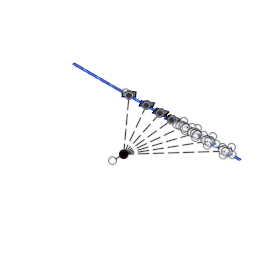
Sonar_bracket_alignment_thingy v7 (Autodesk Fusion 360 design; units mm, degrees)
Autodesk Fusion 360 part; units mm, degrees
note: some values were not read from the file. Set by a fixed rule: which sketch regions a step uses.
sketch "Sketch1" plane through (0, 0, 0) normal (0, 1, 0) x (1, 0, 0)
  line L0 (0, 0) -> (31.2124, 296.9662) construction
  line L1 (0, 0) -> (96.3772, 296.6185) construction
  line L2 (0, 0) -> (170.86, 295.9383) construction
  line L3 (0, 0) -> (265.5789, 294.9552) construction
  line L4 (0, 0) -> (0, -60) construction
  line L5 (0, 0) -> (-31.2124, 296.9662) construction
  line L6 (0, 0) -> (-170.86, 295.9383) construction
  line L7 (0, 0) -> (-265.5789, 294.9552) construction
  line L8 (0, 0) -> (-96.3772, 296.6185) construction
  line L9 (-257.5953, 325.6922) -> (-296.982, 290.2283)
  line L10 (-296.982, 290.2283) -> (-273.5624, 264.2182)
  line L11 (-273.5624, 264.2182) -> (-234.1758, 299.6822)
  line L12 (-234.1758, 299.6822) -> (-257.5953, 325.6922)
  line L13 (-257.5953, 325.6922) -> (-273.5624, 264.2182) construction
  line L14 (-296.982, 290.2283) -> (-234.1758, 299.6822) construction
  line L15 (-156.6604, 324.3437) -> (-202.5597, 297.8437)
  line L16 (-202.5597, 297.8437) -> (-185.0597, 267.5328)
  line L17 (-185.0597, 267.5328) -> (-139.1604, 294.0328)
  line L18 (-139.1604, 294.0328) -> (-156.6604, 324.3437)
  line L19 (-156.6604, 324.3437) -> (-185.0597, 267.5328) construction
  line L20 (-76.582, 321.451) -> (-126.988, 305.0731)
  line L21 (-126.988, 305.0731) -> (-116.1724, 271.7861)
  line L22 (-116.1724, 271.7861) -> (-65.7664, 288.164)
  line L23 (-65.7664, 288.164) -> (-76.582, 321.451)
  line L24 (-76.582, 321.451) -> (-116.1724, 271.7861) construction
  line L25 (-126.988, 305.0731) -> (-65.7664, 288.164) construction
  line L26 (-6.6868, 317.1404) -> (-59.3965, 311.6004)
  line L27 (-59.3965, 311.6004) -> (-55.738, 276.7921)
  line L28 (-55.738, 276.7921) -> (-3.0283, 282.3321)
  line L29 (-3.0283, 282.3321) -> (-6.6868, 317.1404)
  line L30 (-6.6868, 317.1404) -> (-55.738, 276.7921) construction
  line L31 (-59.3965, 311.6004) -> (-3.0283, 282.3321) construction
  line L32 (3.0283, 282.3321) -> (6.6868, 317.1404)
  line L33 (6.6868, 317.1404) -> (59.3965, 311.6004)
  line L34 (55.738, 276.7921) -> (3.0283, 282.3321)
  line L35 (59.3965, 311.6004) -> (55.738, 276.7921)
  line L36 (116.1724, 271.7861) -> (65.7664, 288.164)
  line L37 (65.7664, 288.164) -> (76.582, 321.451)
  line L38 (76.582, 321.451) -> (126.988, 305.0731)
  line L39 (126.988, 305.0731) -> (116.1724, 271.7861)
  line L40 (139.1604, 294.0328) -> (156.6604, 324.3437)
  line L41 (156.6604, 324.3437) -> (202.5597, 297.8437)
  line L42 (202.5597, 297.8437) -> (185.0597, 267.5328)
  line L43 (185.0597, 267.5328) -> (139.1604, 294.0328)
  line L44 (273.5624, 264.2182) -> (234.1758, 299.6822)
  line L45 (234.1758, 299.6822) -> (257.5953, 325.6922)
  line L46 (257.5953, 325.6922) -> (296.982, 290.2283)
  line L47 (296.982, 290.2283) -> (273.5624, 264.2182)
  line L48 (-258.5243, 324.8558) -> (-296.0531, 291.0647)
  line L49 (-296.0531, 291.0647) -> (-272.6335, 265.0547)
  line L50 (-272.6335, 265.0547) -> (-235.1047, 298.8457)
  line L51 (-235.1047, 298.8457) -> (-258.5243, 324.8558)
  line L52 (-258.5243, 324.8558) -> (-272.6335, 265.0547) construction
  line L53 (-296.0531, 291.0647) -> (-235.1047, 298.8457) construction
  line L54 (-157.7429, 323.7187) -> (-201.4772, 298.4687)
  line L55 (-201.4772, 298.4687) -> (-183.9772, 268.1578)
  line L56 (-183.9772, 268.1578) -> (-140.2429, 293.4078)
  line L57 (-140.2429, 293.4078) -> (-157.7429, 323.7187)
  line L58 (-157.7429, 323.7187) -> (-183.9772, 268.1578) construction
  line L59 (-201.4772, 298.4687) -> (-140.2429, 293.4078) construction
  line L60 (-77.7708, 321.0647) -> (-125.7992, 305.4593)
  line L61 (-125.7992, 305.4593) -> (-114.9836, 272.1724)
  line L62 (-114.9836, 272.1724) -> (-66.9552, 287.7777)
  line L63 (-66.9552, 287.7777) -> (-77.7708, 321.0647)
  line L64 (-77.7708, 321.0647) -> (-114.9836, 272.1724) construction
  line L65 (-125.7992, 305.4593) -> (-66.9552, 287.7777) construction
  line L66 (-7.93, 317.0097) -> (-58.1533, 311.731)
  line L67 (-58.1533, 311.731) -> (-54.4948, 276.9228)
  line L68 (-54.4948, 276.9228) -> (-4.2715, 282.2015)
  line L69 (-4.2715, 282.2015) -> (-7.93, 317.0097)
  line L70 (-7.93, 317.0097) -> (-54.4948, 276.9228) construction
  line L71 (-58.1533, 311.731) -> (-4.2715, 282.2015) construction
  line L72 (296.0531, 291.0647) -> (272.6335, 265.0547)
  line L73 (235.1047, 298.8457) -> (258.5243, 324.8558)
  line L74 (201.4772, 298.4687) -> (183.9772, 268.1578)
  line L75 (140.2429, 293.4078) -> (157.7429, 323.7187)
  line L76 (125.7992, 305.4593) -> (114.9836, 272.1724)
  line L77 (66.9552, 287.7777) -> (77.7708, 321.0647)
  line L78 (58.1533, 311.731) -> (54.4948, 276.9228)
  line L79 (4.2715, 282.2015) -> (7.93, 317.0097)
  line L80 (340.5789, 293.5101) -> (-559.4211, 293.5101)
  line L81 (-559.4211, 293.5101) -> (-559.4211, 284.5101)
  line L82 (-559.4211, 284.5101) -> (340.5789, 284.5101)
  line L83 (340.5789, 284.5101) -> (340.5789, 293.5101)
  line L84 (340.5789, 293.5101) -> (-559.4211, 284.5101) construction
  line L85 (-559.4211, 293.5101) -> (340.5789, 284.5101) construction
  line L86 (-257.6212, 293.5101) -> (-282.6212, 293.5101)
  line L87 (-559.4211, 289.0101) -> (340.5789, 289.0101) construction
  circle A0 centre (-260.2258, 289.0101) radius 3.5
  line L88 (-272.7258, 293.5101) -> (-247.7258, 293.5101)
  line L89 (-247.7258, 293.5101) -> (-247.7258, 284.5101)
  line L90 (-247.7258, 284.5101) -> (-272.7258, 284.5101)
  line L91 (-272.7258, 284.5101) -> (-272.7258, 293.5101)
  line L92 (-272.7258, 293.5101) -> (-247.7258, 284.5101) construction
  line L93 (-247.7258, 293.5101) -> (-272.7258, 284.5101) construction
  circle A1 centre (-166.86, 289.0101) radius 3.5
  line L94 (-179.36, 293.5101) -> (-154.36, 293.5101)
  line L95 (-154.36, 293.5101) -> (-154.36, 284.5101)
  line L96 (-154.36, 284.5101) -> (-179.36, 284.5101)
  line L97 (-179.36, 284.5101) -> (-179.36, 293.5101)
  line L98 (-179.36, 293.5101) -> (-154.36, 284.5101) construction
  line L99 (-154.36, 293.5101) -> (-179.36, 284.5101) construction
  circle A2 centre (-93.9051, 289.0101) radius 3.5
  line L100 (-106.4051, 293.5101) -> (-81.4051, 293.5101)
  line L101 (-81.4051, 293.5101) -> (-81.4051, 284.5101)
  line L102 (-81.4051, 284.5101) -> (-106.4051, 284.5101)
  line L103 (-106.4051, 284.5101) -> (-106.4051, 293.5101)
  line L104 (-106.4051, 293.5101) -> (-81.4051, 284.5101) construction
  line L105 (-81.4051, 293.5101) -> (-106.4051, 284.5101) construction
  circle A3 centre (-30.3762, 289.0101) radius 3.5
  line L106 (-42.8762, 293.5101) -> (-17.8762, 293.5101)
  line L107 (-17.8762, 293.5101) -> (-17.8762, 284.5101)
  line L108 (-17.8762, 284.5101) -> (-42.8762, 284.5101)
  line L109 (-42.8762, 284.5101) -> (-42.8762, 293.5101)
  line L110 (-42.8762, 293.5101) -> (-17.8762, 284.5101) construction
  line L111 (-17.8762, 293.5101) -> (-42.8762, 284.5101) construction
  line L112 (17.8762, 293.5101) -> (17.8762, 284.5101)
  circle A4 centre (30.3762, 289.0101) radius 3.5
  line L113 (42.8762, 284.5101) -> (42.8762, 293.5101)
  line L114 (81.4051, 293.5101) -> (81.4051, 284.5101)
  circle A5 centre (93.9051, 289.0101) radius 3.5
  line L115 (106.4051, 284.5101) -> (106.4051, 293.5101)
  line L116 (154.36, 293.5101) -> (154.36, 284.5101)
  line L117 (179.36, 284.5101) -> (179.36, 293.5101)
  circle A6 centre (166.86, 289.0101) radius 3.5
  line L118 (247.7258, 293.5101) -> (247.7258, 284.5101)
  line L119 (272.7258, 284.5101) -> (272.7258, 293.5101)
  circle A7 centre (260.2258, 289.0101) radius 3.5
  point P0 (-265.5789, 294.9552)
  point P1 (-170.86, 295.9383)
  point P2 (-96.3772, 296.6185)
  point P3 (-31.2124, 296.9662)
  point P4 (-265.5789, 294.9552)
  point P5 (-170.86, 295.9383)
  point P6 (-96.3772, 296.6185)
  point P7 (-31.2124, 296.9662)
  point P8 (-265.5789, 294.9552)
  point P9 (-170.86, 295.9383)
  point P10 (-96.3772, 296.6185)
  point P11 (-31.2124, 296.9662)
  point P12 (-260.2258, 289.0101)
  point P13 (-166.86, 289.0101)
  point P14 (-93.9051, 289.0101)
  point P15 (-30.3762, 289.0101)
  dimension "d2" = 12
  dimension "d3" = 12
  dimension "d4" = 12
  dimension "d5" = 12
  dimension "d9" = 35
  dimension "d10" = 35
  dimension "d11" = 35
  dimension "d15" = 35
  dimension "d16" = 53
  dimension "d17" = 53
  dimension "d18" = 53
  dimension "d20" = 53
  dimension "d41" = 50.5
  dimension "d42" = 50.5
  dimension "d43" = 50.5
  dimension "d44" = 50.5
  dimension "d62" = 9
  dimension "d63" = 75
  dimension "d85" = 25
  dimension "d86" = 7
  dimension "d87" = 9.5
  dimension "d88" = 900
  dimension "d89" = 9.5
  dimension "d90" = 7
  dimension "d91" = 25
  dimension "d92" = 7
  dimension "d93" = 25
  dimension "d94" = 9.5
  dimension "d95" = 25
  dimension "d96" = 7
  dimension "d97" = 9.5
  constraint coincident L0.start L1.start
  constraint vertical L4
  constraint symmetric L0.start L4 L1.start
  constraint symmetric L0.end L4 P11
  constraint symmetric L1.end L4 P10
  constraint symmetric L2.end L4 P5
  constraint symmetric L3.end L4 P8
  constraint perpendicular L9 L10
  constraint parallel L9 L11
  constraint parallel L10 L12
  constraint coincident L13 P8
  constraint coincident L14 P8
  constraint coincident P8 P4
  constraint perpendicular L15 L16
  constraint parallel L15 L17
  constraint parallel L16 L18
  constraint coincident L19 P9
  constraint coincident P5 P1
  constraint perpendicular L20 L21
  constraint parallel L20 L22
  constraint parallel L21 L23
  constraint coincident L24 P10
  constraint coincident L25 P10
  constraint coincident P10 P6
  constraint perpendicular L26 L27
  constraint parallel L26 L28
  constraint parallel L27 L29
  constraint coincident L30 P11
  constraint coincident L31 P11
  constraint coincident P11 P7
  constraint perpendicular L7 L11
  constraint perpendicular L6 L17
  constraint perpendicular L8 L22
  constraint perpendicular L5 L28
  constraint symmetric L4 L9.start L45.end
  constraint symmetric L4 L9.end L46.end
  constraint symmetric L4 L10.end L44.start
  constraint symmetric L4 L11.end L44.end
  constraint symmetric L4 L15.start L40.end
  constraint symmetric L4 L15.end L41.end
  constraint symmetric L4 L16.end L42.end
  constraint symmetric L4 L17.end L40.start
  constraint symmetric L4 L20.start L37.end
  constraint symmetric L4 L20.end L38.end
  constraint symmetric L4 L21.end L36.start
  constraint symmetric L4 L22.end L36.end
  constraint symmetric L4 L26.start L32.end
  constraint symmetric L4 L26.end L33.end
  constraint symmetric L4 L27.end L34.start
  constraint symmetric L4 L28.end L32.start
  constraint perpendicular L48 L49
  constraint parallel L48 L50
  constraint parallel L49 L51
  constraint coincident L52 P8
  constraint coincident L53 P8
  constraint perpendicular L54 L55
  constraint parallel L54 L56
  constraint parallel L55 L57
  constraint coincident L58 P9
  constraint coincident L59 P9
  constraint perpendicular L60 L61
  constraint parallel L60 L62
  constraint parallel L61 L63
  constraint coincident L64 P10
  constraint coincident L65 P10
  constraint perpendicular L66 L67
  constraint parallel L66 L68
  constraint parallel L67 L69
  constraint coincident L70 P11
  constraint coincident L71 P11
  constraint collinear L26 L66
  constraint collinear L20 L60
  constraint collinear L15 L54
  constraint collinear L9 L48
  constraint symmetric L4 L48.start L73.end
  constraint symmetric L4 L48.end L72.start
  constraint symmetric L4 L49.end L72.end
  constraint symmetric L4 L50.end L73.start
  constraint symmetric L4 L54.start L75.end
  constraint symmetric L4 L54.end L74.start
  constraint symmetric L4 L55.end L74.end
  constraint symmetric L4 L56.end L75.start
  constraint symmetric L4 L60.start L77.end
  constraint symmetric L4 L60.end L76.start
  constraint symmetric L4 L61.end L76.end
  constraint symmetric L4 L62.end L77.start
  constraint symmetric L4 L66.start L79.end
  constraint symmetric L4 L66.end L78.start
  constraint symmetric L4 L67.end L78.end
  constraint symmetric L4 L68.end L79.start
  constraint perpendicular L80 L81
  constraint parallel L80 L82
  constraint parallel L81 L83
  constraint horizontal L80
  constraint horizontal L86
  constraint coincident L80 L86.start
  constraint horizontal L87
  constraint symmetric L80 L82 L87
  constraint coincident L81 L87.start
  constraint coincident L83 L87.end
  constraint coincident L87 P12
  constraint coincident L7 P12
  constraint perpendicular L88 L89
  constraint parallel L88 L90
  constraint parallel L89 L91
  constraint horizontal L88
  constraint coincident L86 L88.start
  constraint coincident L92 P12
  constraint coincident L93 P12
  constraint coincident P12 A0.centre
  constraint coincident L11 L50.end
  constraint coincident L87 P13
  constraint coincident L6 P13
  constraint perpendicular L94 L95
  constraint parallel L94 L96
  constraint parallel L95 L97
  constraint horizontal L94
  constraint coincident L98 P13
  constraint coincident L99 P13
  constraint coincident P13 A1.centre
  constraint coincident L80 L94.start
  constraint coincident L17 L56.end
  constraint perpendicular L100 L101
  constraint parallel L100 L102
  constraint parallel L101 L103
  constraint horizontal L100
  constraint coincident L80 L100.start
  constraint coincident L104 P14
  constraint coincident L105 P14
  constraint coincident P14 A2.centre
  constraint coincident L8 P14
  constraint coincident L87 P14
  constraint perpendicular L106 L107
  constraint parallel L106 L108
  constraint parallel L107 L109
  constraint horizontal L106
  constraint coincident L80 L106.start
  constraint coincident L110 P15
  constraint coincident L111 P15
  constraint coincident P15 A3.centre
  constraint coincident L87 P15
  constraint coincident L5 P15
  constraint symmetric L4 A0 A7
  constraint symmetric L4 L88.start L119.end
  constraint symmetric L4 L88.end L118.start
  constraint symmetric L4 L89.end L118.end
  constraint symmetric L4 L90.end L119.start
  constraint symmetric L4 A1 A6
  constraint symmetric L4 L94.start L117.end
  constraint symmetric L4 L94.end L116.start
  constraint symmetric L4 L95.end L116.end
  constraint symmetric L4 L96.end L117.start
  constraint symmetric L4 A2 A5
  constraint symmetric L4 L100.start L115.end
  constraint symmetric L4 L100.end L114.start
  constraint symmetric L4 L101.end L114.end
  constraint symmetric L4 L102.end L115.start
  constraint symmetric L4 A3 A4
  constraint symmetric L4 L106.start L113.end
  constraint symmetric L4 L106.end L112.start
  constraint symmetric L4 L107.end L112.end
  constraint symmetric L4 L108.end L113.start
  measures "d2" angle of L2 L3
  measures "d3" angle of L1 L2
  measures "d4" angle of L0 L1
  measures "d5" angle of L0 L5
  measures "d9" distance of L9.start L11.end
  measures "d10" distance of L15.start L17.end
  measures "d11" distance of L20.start L22.end
  measures "d15" distance of L26.start L28.end
  measures "d16" distance of L9.start L9.end
  measures "d17" distance of L15.start L15.end
  measures "d18" distance of L20.start L20.end
  measures "d20" distance of L26.start L26.end
  measures "d41" distance of L67 L69
  measures "d42" distance of L55 L57
  measures "d43" distance of L61 L63
  measures "d44" distance of L49 L51
  measures "d62" distance of L80 L82
  measures "d63" distance of L3.end L83
  measures "d85" distance of L89 L91
  measures "d86" diameter of A0
  measures "d87" distance of L11 P12
  measures "d88" distance of L80.start L80.end
  measures "d89" distance of L56 P13
  measures "d90" diameter of A1
  measures "d91" distance of L95 L97
  measures "d92" diameter of A2
  measures "d93" distance of L100.start L100.end
  measures "d94" distance of L62 P14
  measures "d95" distance of L107.end L108.end
  measures "d96" diameter of A3
  measures "d97" distance of L28 P15
extrude "Extrude1" add sketch "Sketch1" along normal blind 2 contours L9 L11 L12 L51 | L9 L11 L48 L50 L51 L80 L86 L88 | L9 L48 L49 L80 L82 L86 L91 | L9 L10 L49 L82 | L11 L50 L80 L89 | L11 L49 L50 L82 L90 | L10 L11 L49 L82 | L11 L50 L80 L82 L86 L88 L89 L90 L91 | A0 makes body 1 in component "Mount1"
extrude "Extrude1'" add sketch "Sketch1" along normal blind 2 separate body contours L16 L55 L80 L82 | L15 L16 L55 L80 | L16 L17 L55 L82 | L55 L80 L82 L97 | L15 L54 L55 L57 L80 L94 | L17 L55 L56 L82 L96 | L17 L56 L80 L82 L94 L95 L96 L97 | L15 L17 L18 L57 L80 | L17 L56 L57 L80 L95 | L17 L57 L80 | A1 makes body 2 in component "Mount2"
extrude "Extrude1''" add sketch "Sketch1" along normal blind 2 separate body contours L21 L61 L80 L82 | L20 L21 L61 L80 | L21 L22 L61 L82 | L61 L80 L82 L103 | L20 L60 L61 L63 L80 L100 | L22 L61 L62 L82 L102 | L80 L82 L100 L101 L102 L103 | L20 L23 L63 L80 | L22 L62 L63 L80 L82 L101 | L22 L23 L63 L80 | A2 makes body 3 in component "Mount3"
extrude "Extrude1'''" add sketch "Sketch1" along normal blind 2 separate body contours L27 L28 L67 L82 | L27 L67 L80 L82 | L26 L27 L67 L80 | L28 L67 L68 L69 L82 L108 | L67 L80 L82 L109 | L26 L66 L67 L69 L80 L106 | L80 L82 L106 L107 L108 L109 | L28 L29 L69 L82 | L69 L80 L82 L107 | L26 L29 L69 L80 | L29 L69 L80 L82 | A3 makes body 4 in component "Mount4"
extrude "Extrude1''''" add sketch "Sketch1" along normal blind 2 separate body contours L32 L34 L79 L82 | L32 L79 L80 L82 | L32 L33 L79 L80 | L34 L78 L79 L82 | L79 L80 L82 L112 | L33 L78 L79 L80 | L80 L82 L112 L113 | L34 L35 L78 L82 | L78 L80 L82 L113 | L33 L35 L78 L80 | L35 L78 L80 L82 | A4 makes body 5 in component "Mount5"
extrude "Extrude1'''''" add sketch "Sketch1" along normal blind 2 separate body contours L36 L76 L82 | L36 L77 L80 L82 L114 | L36 L37 L77 L80 | L37 L38 L77 L80 | L36 L39 L76 L82 | L80 L82 L114 L115 | L38 L76 L77 L80 | L76 L80 L82 L115 | L39 L76 L80 L82 | L38 L39 L76 L80 | A5 makes body 6 in component "Mount6"
extrude "Extrude1''''''" add sketch "Sketch1" along normal blind 2 separate body contours L43 L75 L80 | L40 L41 L43 L75 L80 | L43 L74 L82 | L43 L80 L82 L116 L117 | L43 L75 L80 L116 | L41 L74 L75 L80 | L42 L43 L74 L82 | L74 L80 L82 L117 | L42 L74 L80 L82 | L41 L42 L74 L80 | A6 makes body 7 in component "Mount7"
extrude "Extrude1'''''''" add sketch "Sketch1" along normal blind 2 separate body contours L44 L80 L118 | L44 L46 L73 L80 | L44 L72 L82 | L44 L80 L82 L118 L119 | L44 L45 L46 L73 | L44 L47 L72 L82 | L46 L72 L80 L82 L119 | L46 L47 L72 L82 | A7 makes body 8 in component "Mount8"
extrude "Extrude3" add sketch "Sketch1" against normal blind 2 separate body contours L9 L11 L12 L51 | L9 L10 L49 L82 | L10 L11 L49 L82 makes body 9 at (-288.2466, -0.6667, -282.3947) makes body 10 at (-241.9823, -0.6667, -308.3522) in component "Mount1"
extrude "Extrude2" add sketch "Sketch1" against normal blind 2 separate body contours L16 L55 L80 L82 | L15 L16 L55 L80 | L16 L17 L55 L82 | L15 L17 L18 L57 L80 | L17 L57 L80 makes body 11 at (-196.7264, -0.6667, -287.7401) makes body 12 at (-144.9937, -0.6667, -304.1365) in component "Mount2"
extrude "Extrude2'" add sketch "Sketch1" against normal blind 2 separate body contours L21 L61 L80 L82 | L20 L21 L61 L80 | L21 L22 L61 L82 | L20 L23 L63 L80 | L22 L23 L63 L80 makes body 13 at (-123.3828, -0.6667, -293.9774) makes body 14 at (-69.3716, -0.6667, -299.2596) in component "Mount3"
extrude "Extrude2''" add sketch "Sketch1" against normal blind 2 separate body contours L27 L28 L67 L82 | L27 L67 L80 L82 | L26 L27 L67 L80 | L28 L29 L69 L82 | L26 L29 L69 L80 | L29 L69 L80 L82 makes body 15 at (-56.9338, -0.6667, -300.1283) makes body 16 at (-4.2478, -0.6667, -293.9349) in component "Mount4"
extrude "Extrude2'''" add sketch "Sketch1" against normal blind 2 separate body contours L32 L34 L79 L82 | L32 L79 L80 L82 | L32 L33 L79 L80 | L34 L35 L78 L82 | L33 L35 L78 L80 | L35 L78 L80 L82 makes body 17 at (56.9338, -0.6667, -300.1283) makes body 18 at (4.2478, -0.6667, -293.9349) in component "Mount5"
extrude "Extrude2''''" add sketch "Sketch1" against normal blind 2 separate body contours L36 L37 L77 L80 | L37 L38 L77 L80 | L36 L39 L76 L82 | L39 L76 L80 L82 | L38 L39 L76 L80 makes body 19 at (69.3716, -0.6667, -299.2596) makes body 20 at (123.3828, -0.6667, -293.9774) in component "Mount6"
extrude "Extrude2'''''" add sketch "Sketch1" against normal blind 2 separate body contours L43 L75 L80 | L40 L41 L43 L75 L80 | L42 L43 L74 L82 | L42 L74 L80 L82 | L41 L42 L74 L80 makes body 21 at (144.9937, -0.6667, -304.1365) makes body 22 at (196.7264, -0.6667, -287.7401) in component "Mount7"
extrude "Extrude2''''''" add sketch "Sketch1" against normal blind 2 separate body contours L44 L45 L46 L73 | L44 L47 L72 L82 | L46 L47 L72 L82 makes body 23 at (288.2466, -1.3333, -282.3947) makes body 24 at (242.9112, -0.6667, -307.5158) in component "Mount8"
extrude "Extrude3'" add sketch "Sketch1" along normal blind 6 separate body contours L27 L67 L80 L82 | L67 L80 L82 L109 | L69 L80 L82 L107 | L29 L69 L80 L82 makes body 25 at (-8.4455, 0, -287.5101) makes body 26 at (-52.3068, 0, -290.5101) in component "Mount4"
extrude "Extrude5" add sketch "Sketch1" along normal blind 6 separate body contours L9 L48 L49 L80 L82 L86 L91 | L9 L10 L49 L82 | L11 L50 L80 L89 makes body 27 at (-285.9655, 0, -290.5101) makes body 28 at (-245.4941, 4, -289.4911) in component "Mount1"
extrude "Extrude6" cut sketch "Sketch1" along normal blind 2 contours A0 bodies 1 in component "Mount1"
extrude "Extrude6'" add sketch "Sketch1" along normal blind 6 separate body contours L16 L55 L80 L82 | L55 L80 L82 L97 | L17 L56 L57 L80 L95 makes body 29 at (-191.4264, 0, -290.5101) makes body 30 at (-149.6543, 2, -287.9741) in component "Mount2"
extrude "Extrude7" cut sketch "Sketch1" along normal blind 2 contours A1 bodies 2 in component "Mount2"
extrude "Extrude4" add sketch "Sketch1" along normal blind 6 separate body contours L21 L61 L80 L82 | L61 L80 L82 L103 | L22 L62 L63 L80 L82 L101 | L22 L23 L63 L80 makes body 31 at (-116.6476, 0, -290.5101) makes body 32 at (-75.3068, 0, -290.5101) in component "Mount3"
extrude "Extrude5'" cut sketch "Sketch1" along normal blind 2 contours A2 bodies 3 in component "Mount3"
extrude "Extrude4'" cut sketch "Sketch1" along normal blind 2 contours A3 bodies 4 in component "Mount4"
extrude "Extrude4''" add sketch "Sketch1" along normal blind 6 separate body contours L32 L79 L80 L82 | L79 L80 L82 L112 | L78 L80 L82 L113 | L35 L78 L80 L82 makes body 33 at (8.4455, 0, -287.5101) makes body 34 at (52.3068, 0, -290.5101) in component "Mount5"
extrude "Extrude5''" cut sketch "Sketch1" along normal blind 2 contours A4 bodies 5 in component "Mount5"
extrude "Extrude4'''" add sketch "Sketch1" along normal blind 6 separate body contours L36 L77 L80 L82 L114 | L36 L37 L77 L80 | L76 L80 L82 L115 | L39 L76 L80 L82 makes body 35 at (75.3068, 0, -290.5101) makes body 36 at (116.6476, 0, -290.5101) in component "Mount6"
extrude "Extrude5'''" cut sketch "Sketch1" along normal blind 2 contours A5 bodies 6 in component "Mount6"
extrude "Extrude4''''" add sketch "Sketch1" along normal blind 6 separate body contours L43 L75 L80 | L43 L75 L80 L116 | L74 L80 L82 L117 | L42 L74 L80 L82 makes body 37 at (149.5953, 2, -288.0082) makes body 38 at (191.4264, 0, -290.5101) in component "Mount7"
extrude "Extrude5''''" cut sketch "Sketch1" along normal blind 2 contours A6 bodies 7 in component "Mount7"
extrude "Extrude4'''''" add sketch "Sketch1" along normal blind 6 separate body contours L44 L80 L118 | L46 L72 L80 L82 L119 | L46 L47 L72 L82 makes body 39 at (245.4941, 2, -289.4911) makes body 40 at (285.9655, 0, -290.5101) in component "Mount8"
extrude "Extrude5'''''" cut sketch "Sketch1" along normal blind 2 contours A7 bodies 8 in component "Mount8"
component "Mount1" placed x (1, 0, 0) y (0, 1, 0) z (0, 0, 1) at (0, 0, 0)
component "Mount2" placed x (1, 0, 0) y (0, 1, 0) z (0, 0, 1) at (0, 0, 0)
component "Mount3" placed x (1, 0, 0) y (0, 1, 0) z (0, 0, 1) at (0, 0, 0)
component "Mount4" placed x (1, 0, 0) y (0, 1, 0) z (0, 0, 1) at (0, 0, 0)
component "Mount5" placed x (1, 0, 0) y (0, 1, 0) z (0, 0, 1) at (0, 0, 0)
component "Mount6" placed x (1, 0, 0) y (0, 1, 0) z (0, 0, 1) at (0, 0, 0)
component "Mount7" placed x (1, 0, 0) y (0, 1, 0) z (0, 0, 1) at (0, 0, 0)
component "Mount8" placed x (1, 0, 0) y (0, 1, 0) z (0, 0, 1) at (0, 0, 0)
equation "alpha = 12 deg"
equation "d2 = alpha"
equation "d3 = alpha"
equation "d4 = alpha"
equation "d5 = alpha"
